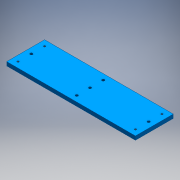
# Autodesk Inventor part: xyStageStilt_pt2
Saved by Autodesk Inventor 2016 (Build 200138000, 138)
## iProperties
Created: 2016-03-18
Part Number: xyStageStilt_pt2
Material: Generic
Document SubType Name: Modeling
Designer: sims01
Density: 1 g/cm^3
Appearance: Default
Author: sims01
Autodesk Inventor part; units mm, degrees
ref_plane "YZ Plane" through (0, 0, 0) normal (1, 0, 0) x (0, 1, 0)
ref_plane "XZ Plane" through (0, 0, 0) normal (0, 1, 0) x (-1, 0, 0)
ref_plane "XY Plane" through (0, 0, 0) normal (0, 0, 1) x (1, 0, 0)
sketch "Sketch1" plane through (0, 0, 0) normal (0, 0, 1) x (1, 0, 0)
  line L0 (-170, 50) -> (170, 50)
  line L1 (170, 50) -> (170, -50)
  line L2 (170, -50) -> (-170, -50)
  line L3 (-170, -50) -> (-170, 50)
  point P0 (0, 0)
  dimension "d0" = 340
  dimension "d1" = 170
  dimension "d2" = 100
  dimension "d3" = 50
  constraints: 8 end point, 2 parallel, 1 horizontal, 1 perpendicular
  measures "d0" distance of L0.start L0.end
  measures "d1" distance from line of L1 point (0, 0)
  measures "d2" distance of L0.end L1.end
  measures "d3" distance from line of point (0, 0) L0
extrude "baseExtrusion" add sketch "Sketch1" along normal blind 10
sketch "Sketch2" plane through (0, 0, 10) normal (0, 0, 1) x (1, 0, 0)
  line L0 (170, 50) -> (-170, 50) projected
  line L1 (-170, 50) -> (-170, -50) projected
  point P0 (0, 0)
  point P1 (-155, 35)
  dimension "d6" = 15
  dimension "d7" = 15
  measures "d6" distance from line of L0 point (-155, 35)
  measures "d7" distance from line of L1 point (-155, 35)
hole "xyStiltpt1m6MountingHoles" at (-155, 35, 10) direction (0, 0, -1) diameter 4.917 end through all thread size "M6x1" class "6H" standard "ISO Metric profile"
mirror "Mirror2" about plane through (0, 0, 0) normal (1, 0, 0) of "xyStiltpt1m6MountingHoles"
mirror "Mirror3" about plane through (0, 0, 0) normal (0, 1, 0) of "xyStiltpt1m6MountingHoles", "Mirror2"
sketch "Sketch4" plane through (0, 0, 0) normal (0, 0, -1) x (-1, 0, 0)
  line L0 (170, -50) -> (170, 50) projected
  line L1 (170, 50) -> (-170, 50) projected
  line L2 (-170, 50) -> (-170, -50) projected
  line L3 (-170, -50) -> (170, -50) projected
  point P0 (0, 0)
  point P1 (155, 0)
  point P2 (0, 0)
  point P3 (0, 35)
  point P4 (0, -35)
  point P5 (-155, 0)
  dimension "d24" = 15
  dimension "d25" = 15
  dimension "d26" = 15
  dimension "d27" = 15
  constraints: 2 coincident, 2 horizontal alignment, 2 vertical alignment
  measures "d24" distance from line of L0 point (155, 0)
  measures "d25" distance from line of L1 point (0, 35)
  measures "d26" distance from line of L2 point (-155, 0)
  measures "d27" distance from line of L3 point (0, -35)
hole "Hole3" at (-155, 0, 0) at (0, 0, 0) at (0, 35, 0) at (0, -35, 0) at (155, 0, 0) direction (0, 0, 1) diameter 6.6 end through all counterbore diameter 18 counterbore depth 4.8 clearance for "Hex Head Cap Screw ISO 24017" size "M6" standard "ISO"
equation "\"d1\" = 0.5 * d0"
equation "\"d3\" = 0.5 * d2"
body "Solid1"
